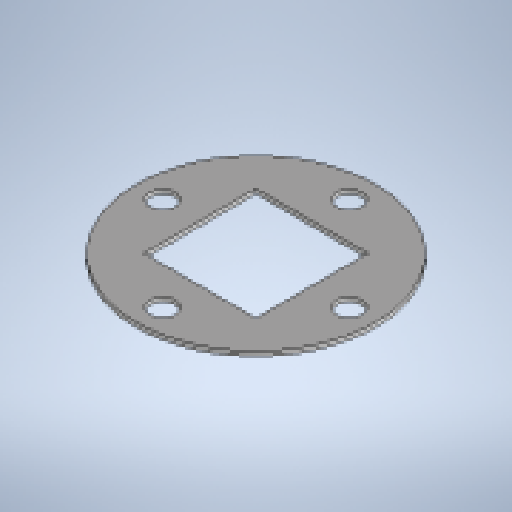
# Autodesk Inventor part: PRS-1651 FDS MAIN  FLANGE_CPY
Saved by Autodesk Inventor 2026.2 (Build 302298010, 298A)
## iProperties
Created: 2025-06-24
Part Number: PRS-1651 FDS MAIN  FLANGE_CPY
Material: Stainless Steel
Document SubType Name: Sheet Metal
Designer: admin
Mass: 326.359 g
Surface Area: 301.648 cm^2
Volume: 40.7948 cm^3
Density: 8 g/cm^3
Flat Pattern Width: 16 cm
Flat Pattern Length: 16 cm
Flat Pattern Area: 256 cm^2
Sheet Metal Rule: Default
Sheet Metal Width: 160,000 mm
Sheet Metal Length: 160,000 mm
Sheet Metal Area: 25600,000 mm^2
Appearance: Default
Author: user
Autodesk Inventor part; units mm, degrees
ref_plane "YZ Plane" through (0, 0, 0) normal (1, 0, 0) x (0, 1, 0)
ref_plane "XZ Plane" through (0, 0, 0) normal (0, 1, 0) x (-1, 0, 0)
ref_plane "XY Plane" through (0, 0, 0) normal (0, 0, 1) x (1, 0, 0)
sketch "Sketch1" plane through (0, 0, 0) normal (0, 0, 1) x (1, 0, 0)
  circle A0 centre (0, 0) radius 80
  line L0 (37.5, 37.5) -> (-37.5, 37.5)
  line L1 (-37.5, 37.5) -> (-37.5, -37.5)
  line L2 (-37.5, -37.5) -> (37.5, -37.5)
  line L3 (37.5, -37.5) -> (37.5, 37.5)
  line L4 (37.5, 37.5) -> (-37.5, -37.5) construction
  line L5 (-37.5, 37.5) -> (37.5, -37.5) construction
  circle A1 centre (0, 0) radius 62.5 construction
  circle A2 centre (-62.5, 0) radius 8.5
  circle A3 centre (0, -62.5) radius 8.5
  circle A4 centre (62.5, 0) radius 8.5
  circle A5 centre (0, 62.5) radius 8.5
  dimension "d171" = 125
  dimension "d157" = 160
  dimension "d158" = 75
  dimension "d176" = 17
  dimension "d179" = 360
  measures "d157" diameter of A0
  measures "d158" distance of L2.end L1.end
  measures "d176" diameter of A2
extrude "Plate5" add sketch "Sketch1" along normal blind 3
body "Solid3"
